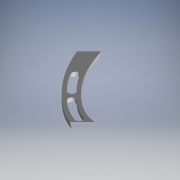
# Autodesk Inventor part: Profile
Saved by Autodesk Inventor 2016 (Build 200138000, 138)
## iProperties
Created: 2015-05-19
Part Number: Profile
Material: Generic
Document SubType Name: Modeling
Designer: Yann
Density: 1 g/cm^3
Appearance: Default
Author: Yann
Autodesk Inventor part; units mm, degrees
ref_plane "YZ Plane" through (0, 0, 0) normal (1, 0, 0) x (0, 1, 0)
ref_plane "XZ Plane" through (0, 0, 0) normal (0, 1, 0) x (-1, 0, 0)
ref_plane "XY Plane" through (0, 0, 0) normal (0, 0, 1) x (1, 0, 0)
sketch "Sketch1" plane through (0, 0, 0) normal (0, 1, 0) x (-1, 0, 0)
  circle A0 centre (0, 0) radius 19.05
  arc A1 (4.4642, 39.1161) -> (-1.9997, -39.3192) centre (0, 0) ccw
  line L0 (-1.9997, -39.3192) -> (49.0185, -41.9138) construction
  line L1 (263.1315, -247.3812) -> (302.3964, -370.4331) construction
  spline S0 degree 4 poles (-1.9997, -39.3192) (49.0185, -41.9138) (105.6374, -72.1982) (173.8913, -120.1961) (263.1315, -247.3812) (302.3964, -370.4331) knots 1 1 1 1 1 1.581444 2 2 2 2 2
  line L2 (4.4642, 39.1161) -> (78.1887, 30.7022) construction
  line L3 (339.9032, -237.0622) -> (377.1456, -345.6975) construction
  spline S1 degree 4 poles (4.4642, 39.1161) (78.1887, 30.7022) (179.8099, -32.9721) (261.2925, -118.1743) (339.9032, -237.0622) (377.1456, -345.6975) knots 0 0 0 0 0 1 2 2 2 2 2
  circle A2 centre (339.9032, -358.4649) radius 19.05
  arc A3 (302.3964, -370.4331) -> (377.1456, -345.6975) centre (339.9032, -358.4649) ccw
  circle A4 centre (339.9032, -358.4649) radius 15.8726 construction
  arc A5 (265.0359, -199.854) -> (201.2966, -118.1743) centre (2.3813, -339.1088) ccw construction
  arc A6 (280.7447, -191.5256) -> (213.1932, -104.9608) centre (2.3813, -339.1088) ccw
  arc A7 (249.3272, -208.1825) -> (189.3999, -131.3879) centre (2.3813, -339.1088) ccw
  arc A8 (249.3272, -208.1825) -> (280.7447, -191.5256) centre (265.0359, -199.854) ccw
  arc A9 (213.1932, -104.9608) -> (189.3999, -131.3879) centre (201.2966, -118.1743) ccw
  arc A10 (161.0182, -77.5529) -> (62.8262, -16.2966) centre (-36.5592, -284.9364) ccw construction
  arc A11 (173.2826, -64.6798) -> (68.9954, 0.3788) centre (-36.5592, -284.9364) ccw
  arc A12 (148.7539, -90.4259) -> (56.657, -32.9721) centre (-36.5592, -284.9364) ccw
  arc A13 (148.7539, -90.4259) -> (173.2826, -64.6798) centre (161.0182, -77.5529) ccw
  arc A14 (68.9954, 0.3788) -> (56.657, -32.9721) centre (62.8262, -16.2966) ccw
  line L4 (78.1887, 30.7022) -> (179.8099, -32.9721) construction
  line L5 (179.8099, -32.9721) -> (261.2925, -118.1743) construction
  line L6 (261.2925, -118.1743) -> (339.9032, -237.0622) construction
  line L7 (49.0185, -41.9138) -> (105.6374, -72.1982) construction
  line L8 (105.6374, -72.1982) -> (173.8913, -120.1961) construction
  line L9 (173.8913, -120.1961) -> (263.1315, -247.3812) construction
  dimension "d0" = 38.1
  dimension "d1" = 20.32
  dimension "d2" = 38.1
  dimension "d3" = 20.32
  dimension "d6" = 17.78
  dimension "d7" = 17.78
  constraints: 25 point on circle, 15 centre point, 12 tangent, 4 coincident, 6 other
  measures "d0" diameter of A0
  measures "d1" radial gap between concentric circles of A3 A2
  measures "d2" diameter of A2
  measures "d3" radial gap between concentric circles of A1 A0
  measures "d6" radial gap between concentric circles of A11 A10
  measures "d7" radial gap between concentric circles of A6 A5
extrude "Extrusion1" add sketch "Sketch1" along normal blind 20
equation "\"d1\" = d3"
equation "\"d2\" = d0"
equation "\"d7\" = d6"
body "Solid1"
